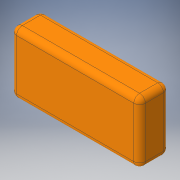
# Autodesk Inventor part: Battery
Saved by Autodesk Inventor 2016 (Build 200138000, 138)
## iProperties
Created: 2016-10-06
Part Number: Battery
Material: Generic
Document SubType Name: Modeling
Designer: desirw
Density: 1 g/cm^3
Appearance: Default
Author: desirw
Autodesk Inventor part; units mm, degrees
ref_plane "YZ Plane" through (0, 0, 0) normal (1, 0, 0) x (0, 1, 0)
ref_plane "XZ Plane" through (0, 0, 0) normal (0, 1, 0) x (-1, 0, 0)
ref_plane "XY Plane" through (0, 0, 0) normal (0, 0, 1) x (1, 0, 0)
sketch "Sketch1" plane through (0, 0, 0) normal (0, 0, 1) x (1, 0, 0)
  line L0 (-7.5576, 4.5871) -> (63.1052, 4.5871)
  line L1 (63.1052, 4.5871) -> (63.1052, -29.4489)
  line L2 (63.1052, -29.4489) -> (-7.5576, -29.4489)
  line L3 (-7.5576, -29.4489) -> (-7.5576, 4.5871)
  point P0 (0, 0)
  dimension "d0" = 70.6628
  dimension "d1" = 34.036
  constraints: 8 end point, 2 parallel, 1 horizontal, 1 perpendicular
  measures "d0" distance of L1.end L2.end
  measures "d1" distance of L0.end L1.end
extrude "Extrusion1" add sketch "Sketch1" along normal blind 16.256
fillet "Fillet1" radius 3.175 12 edges at (27.7738, 4.5871, 16.256) (-7.5576, -12.4309, 16.256) (63.1052, -12.4309, 16.256) (27.7738, -29.4489, 16.256) (27.7738, 4.5871, 0) (27.7738, -29.4489, 0) (63.1052, -12.4309, 0) (-7.5576, -12.4309, 0) (-7.5576, -29.4489, 8.128) (-7.5576, 4.5871, 8.128) (63.1052, 4.5871, 8.128) (63.1052, -29.4489, 8.128)
body "Solid1"
